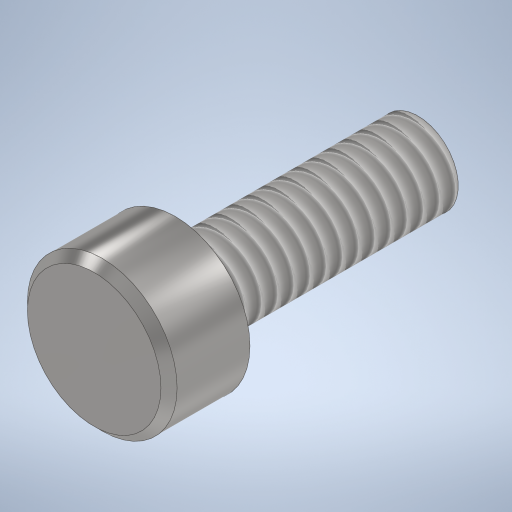
# Autodesk Inventor part: M2×6
Saved by Autodesk Inventor 2024 (Build 280153000, 153)
## iProperties
Created: 2025-06-01
Part Number: M2×6
Material: ステンレス鋼
Document SubType Name: Modeling
Designer: 1412z
Density: 8 g/cm^3
Appearance: 半つや出し
Author: 1412z
Autodesk Inventor part; units mm, degrees
ref_plane "YZ Plane" through (0, 0, 0) normal (1, 0, 0) x (0, 1, 0)
ref_plane "XZ Plane" through (0, 0, 0) normal (0, 1, 0) x (-1, 0, 0)
ref_plane "XY Plane" through (0, 0, 0) normal (0, 0, 1) x (1, 0, 0)
sketch "スケッチ1" plane through (0, 0, 0) normal (0, 0, 1) x (1, 0, 0)
  circle A0 centre (0, 0) radius 1.85
  dimension "d0" = 3.7
  constraints: 1 centre point, 1 coincident
  measures "d0" diameter of A0
extrude "押し出し1" add sketch "スケッチ1" along normal blind 2
sketch "スケッチ2" plane through (0, 0, 0) normal (0, 0, -1) x (-1, 0, 0)
  circle A0 centre (0, 0) radius 1
  dimension "d3" = 2
  constraints: 1 centre point, 1 coincident
  measures "d3" diameter of A0
extrude "押し出し2" add sketch "スケッチ2" along normal blind 6
thread "ねじ1" size "M2x0.4" class "6g" standard "ANSI Metric M Profile" full length
chamfer "面取り1" distance 0.2 angle 45 1 edges at (-1.85, 0, 2)
